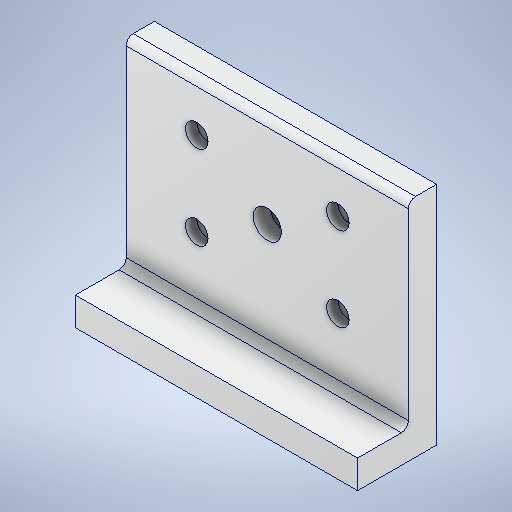
# Autodesk Inventor part: Molde
Saved by Autodesk Inventor 2025.1 (Build 291241000, 241)
## iProperties
Created: 2025-01-29
Part Number: Molde
Material: Aluminum 6061
Document SubType Name: Modeling
Designer: yovan
Mass: 51855.9 g
Surface Area: 6273.43 cm^2
Volume: 19205.9 cm^3
Density: 2.7 g/cm^3
Appearance: Aluminum - Flat
Author: yovan
Autodesk Inventor part; units mm, degrees
ref_plane "YZ Plane" through (0, 0, 0) normal (1, 0, 0) x (0, 1, 0)
ref_plane "XZ Plane" through (0, 0, 0) normal (0, 1, 0) x (-1, 0, 0)
ref_plane "XY Plane" through (0, 0, 0) normal (0, 0, 1) x (1, 0, 0)
sketch "Sketch1" plane through (0, 0, 0) normal (1, 0, 0) x (0, 1, 0)
  line L0 (400, 120) -> (0, 120)
  line L1 (0, 40) -> (0, 62.8571)
  line L2 (400, 120) -> (0, 120)
  line L3 (0, 120) -> (0, 30)
  line L4 (0, 30) -> (400, 30)
  line L5 (400, 30) -> (400, 120)
  dimension "d54" = 400
  dimension "d55" = 90
  constraints: 12 end point, 2 parallel, 1 horizontal, 1 perpendicular
  measures "d54" distance of L0.start L0.end
  measures "d55" distance of L4.end L0.start
extrude "Extrusion1" add sketch "Sketch1" along normal blind 500
sketch "Sketch2" plane through (500, 0, 0) normal (1, 0, 0) x (0, 0, -1)
  line L0 (-30, 400) -> (20, 400)
  line L1 (20, 400) -> (20, 350)
  line L2 (20, 350) -> (-30, 350)
  line L3 (-30, 350) -> (-30, 400)
  arc A0 (-42.5, 0) -> (-30, 12.5) centre (-42.5, 12.5) ccw
  line L4 (-120, 0) -> (-30, 0) projected
  line L5 (-30, 0) -> (-64.3382, 0)
  line L6 (-30, 12.5) -> (-30, 0)
  line L7 (-120, 400) -> (-120, 0) projected
  line L8 (-120, 0) -> (-70, 0)
  line L9 (-70, 0) -> (-70, 40)
  line L10 (-70, 40) -> (-120, 40)
  line L11 (-120, 40) -> (-120, 0)
  point P0 (-120, 40)
  point P1 (-70, 0)
  dimension "d11" = 50
  dimension "d12" = 50
  dimension "d33" = 12.5
  dimension "d38" = 50
  dimension "d39" = 40
  constraints: 20 end point, 4 parallel, 3 horizontal, 2 perpendicular, 2 point on circle, 1 centre point
  measures "d11" distance of L1.end L2.end
  measures "d12" distance of L0.end L1.end
  measures "d33" radius of A0
  measures "d38" distance of L10.end L9.end
  measures "d39" distance of L9.end L8.end
extrude "Extrusion10" cut sketch "Sketch2" against normal blind 100 contours L7 L10 L9 L4
extrude "Extrusion11" cut sketch "Sketch2" against normal blind 500 contours A0 L6 L4
extrude "Extrusion12" add sketch "Sketch2" against normal blind 500 contours L0 L1 L2 L3
sketch "Sketch5" plane through (500, 40, 70) normal (0, -1, 0) x (1, 0, 0)
  line L0 (0, 0) -> (-100, 0) projected
  line L1 (0, 0) -> (-90, 0)
  line L2 (-90, 0) -> (-90, 45)
  line L3 (-90, 45) -> (0, 45)
  line L4 (0, 45) -> (0, 0)
  line L5 (0, 22.5) -> (-30, 22.5)
  circle A0 centre (-30, 22.5) radius 7.5
  line L6 (-30, 22.5) -> (-65, 22.5)
  circle A1 centre (-65, 22.5) radius 7.5
  point P0 (-500, -70)
  dimension "d46" = 90
  dimension "d47" = 45
  dimension "d48" = 30
  dimension "d49" = 15
  dimension "d50" = 35
  dimension "d51" = 15
  constraints: 12 end point, 3 horizontal, 2 centre point, 2 coincident, 2 parallel, 1 midpoint, 1 perpendicular
  measures "d46" distance of L2.end L3.end
  measures "d47" distance of L1.end L2.end
  measures "d48" distance of L5.start L5.end
  measures "d49" diameter of A0
  measures "d50" distance of L6.start L6.end
  measures "d51" diameter of A1
extrude "Extrusion13" cut sketch "Sketch5" against normal blind 10 contours A0 L6 L5 | L5 L6 A0 | A1
fillet "Fillet3" radius 12.5 1 edges at (250, 350, 30)
sketch "Sketch6" plane through (500, 12.5, 30) normal (0, 0, -1) x (-1, 0, 0)
  line L0 (500, 325) -> (500, 337.5) projected
  circle A0 centre (250, 176.25) radius 25
  circle A1 centre (125, 250.625) radius 20
  circle A2 centre (375, 250.625) radius 20
  circle A3 centre (375, 101.875) radius 20
  circle A4 centre (125, 101.875) radius 20
  dimension "d57" = 50
  dimension "d58" = 40
  dimension "d59" = 40
  dimension "d60" = 40
  dimension "d61" = 40
  constraints: 5 centre point
  measures "d57" diameter of A0
  measures "d58" diameter of A1
  measures "d59" diameter of A2
  measures "d60" diameter of A3
  measures "d61" diameter of A4
extrude "Extrusion14" add sketch "Sketch6" along normal blind 30 contours A0
extrude "Extrusion15" add sketch "Sketch6" along normal blind 20 contours A1 | A2 | A3 | A4
sketch "Sketch7" plane through (500, 0, 0) normal (1, 0, 0) x (0, 0, -1)
  line L0 (-50, 0) -> (20, 0)
  line L1 (20, 0) -> (20, 400)
  line L2 (20, 400) -> (-50, 400)
  line L3 (-50, 400) -> (-50, 0)
  constraints: 8 end point, 2 perpendicular, 1 horizontal
extrude "Extrusion16" add sketch "Sketch7" against normal blind 500 separate body
combine bodies "Combine1" operation type subtract main body 2 bodies to subtract 1
sketch "Sketch8" plane through (0, 0, -20) normal (0, -1, 0) x (1, 0, 0)
  line L0 (500, 62.5) -> (0, 62.5)
  line L1 (0, 62.5) -> (0, 0)
  line L2 (0, 0) -> (500, 0)
  line L3 (500, 0) -> (500, 62.5)
  constraints: 8 end point, 2 parallel, 1 horizontal, 1 perpendicular
extrude "Extrusion17" add sketch "Sketch8" along normal blind 50 bodies 2
sketch "Sketch9" plane through (0, 0, 42.5) normal (0, 0, 1) x (1, 0, 0)
  line L0 (500, 0) -> (500, -50) projected
  line L1 (0, 0) -> (500, 0)
  line L2 (500, 0) -> (500, -50)
  line L3 (500, -50) -> (0, -50)
  line L4 (0, -50) -> (0, 0)
  constraints: 8 end point, 2 parallel, 1 horizontal, 1 perpendicular
extrude "Extrusion18" add sketch "Sketch9" along normal blind 77.5 bodies 2
body "Solid2"
